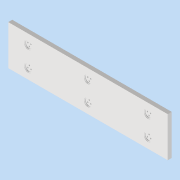
# Autodesk Inventor part: Platt oben
Saved by Autodesk Inventor 2021 (Build 250183000, 183)
## iProperties
Created: 2024-03-13
Part Number: Platt oben
Material: Generic
Document SubType Name: Modeling
Designer: Nokia
Density: 1 g/cm^3
Appearance: Smooth - Ash
Mass: 3100.69 g
Surface Area: 3710.93 cm^2
Volume: 3100.69 cm^3
Author: Nokia
Autodesk Inventor part; units mm, degrees
ref_plane "YZ Plane" through (0, 0, 0) normal (1, 0, 0) x (0, 1, 0)
ref_plane "XZ Plane" through (0, 0, 0) normal (0, 1, 0) x (-1, 0, 0)
ref_plane "XY Plane" through (0, 0, 0) normal (0, 0, 1) x (1, 0, 0)
sketch "Sketch1" plane through (0, 0, 0) normal (0, 0, 1) x (1, 0, 0)
  line L0 (-400, -100) -> (-400, 100)
  line L1 (-400, 100) -> (400, 100)
  line L2 (400, 100) -> (400, -100)
  line L3 (400, -100) -> (-400, -100)
  point P0 (0, 0)
  dimension "d2" = 800
  dimension "d3" = 200
  constraints: 8 end point, 3 perpendicular
  measures "d2" distance of L0.end L1.end
  measures "d3" distance of L1.end L2.end
extrude "Extrusion1" add sketch "Sketch1" along normal blind 20
sketch "Sketch5" plane through (0, 0, 20) normal (0, 0, 1) x (1, 0, 0)
  line L0 (0, 0) -> (0, 50)
  circle A0 centre (0, 50) radius 17
  line L1 (0, 0) -> (-150, 0)
  line L2 (-150, 0) -> (-150, 100)
  line L3 (-400, 100) -> (400, 100)
  circle A1 centre (0, -50) radius 17
  circle A2 centre (-300, 50) radius 17
  circle A3 centre (-300, -50) radius 17
  circle A4 centre (300, 50) radius 17
  circle A5 centre (300, -50) radius 17
  circle A6 centre (0, 50) radius 20
  circle A7 centre (0, -50) radius 20
  circle A8 centre (-300, 50) radius 20
  circle A9 centre (-300, -50) radius 20
  circle A10 centre (300, -50) radius 20
  circle A11 centre (300, 50) radius 20
  dimension "d18" = 50
  dimension "d19" = 34
  dimension "d20" = 150
  dimension "d43" = 40
  constraints: 12 centre point, 10 symmetric about line, 8 end point, 2 coincident, 1 horizontal, 1 perpendicular, 1 point on line, 1 vertical, 10 other
  measures "d18" distance of L0.start L0.end
  measures "d19" diameter of A0
  measures "d20" distance of L0.start L1.end
  measures "d43" diameter of A6
extrude "Extrusion4" cut sketch "Sketch5" against normal blind 6 contours A0 | A1 | A2 | A3 | A4 | A5
sketch "Sketch6" plane through (0, 0, 0) normal (0, 0, -1) x (-1, 0, 0)
  line L0 (0, 0) -> (0, 50)
  circle A0 centre (0, 50) radius 20
  line L1 (0, 0) -> (-150, 0)
  line L2 (-150, 0) -> (-150, 100)
  line L3 (-400, 100) -> (400, 100)
  circle A1 centre (0, -50) radius 20
  circle A2 centre (-300, 50) radius 20
  circle A3 centre (-300, -50) radius 20
  circle A4 centre (300, 50) radius 20
  circle A5 centre (300, -50) radius 20
  circle A6 centre (0, 50) radius 15
  circle A7 centre (0, 41) radius 3.5
  circle A8 centre (7.7942, 54.5) radius 3.5
  circle A9 centre (-7.7942, 54.5) radius 3.5
  circle A10 centre (0, -50) radius 15
  circle A11 centre (0, -41) radius 3.5
  circle A12 centre (7.7942, -54.5) radius 3.5
  circle A13 centre (-7.7942, -54.5) radius 3.5
  circle A14 centre (-300, 50) radius 15
  circle A15 centre (-300, 41) radius 3.5
  circle A16 centre (-307.7942, 54.5) radius 3.5
  circle A17 centre (-292.2058, 54.5) radius 3.5
  circle A18 centre (-307.7942, -54.5) radius 3.5
  circle A19 centre (-300, -41) radius 3.5
  circle A20 centre (-292.2058, -54.5) radius 3.5
  circle A21 centre (-300, -50) radius 15
  circle A22 centre (300, -50) radius 15
  circle A23 centre (292.2058, -54.5) radius 3.5
  circle A24 centre (300, -41) radius 3.5
  circle A25 centre (307.7942, -54.5) radius 3.5
  circle A26 centre (300, 41) radius 3.5
  circle A27 centre (292.2058, 54.5) radius 3.5
  circle A28 centre (307.7942, 54.5) radius 3.5
  circle A29 centre (300, 50) radius 15
  dimension "d23" = 50
  dimension "d24" = 40
  dimension "d25" = 150
  dimension "d28" = 30
  dimension "d30" = 7
  dimension "d33" = 360
  dimension "d42" = 9
  constraints: 30 centre point, 25 symmetric about line, 8 end point, 2 coincident, 1 horizontal, 1 perpendicular, 1 point on line, 1 vertical, 32 other
  measures "d23" distance of L0.start L0.end
  measures "d24" diameter of A0
  measures "d25" distance of L0.start L1.end
  measures "d28" diameter of A6
  measures "d30" diameter of A7
  measures "d42" distance of A7.centre L0.end
extrude "Extrusion5" cut sketch "Sketch6" against normal blind 8 contours A7 L0 | L0 A7 | A0 | A1 | A2 | A3 | A4 | A5 | A6 | A8 | A9 | A10 | A11 | A12 | A13 | A14 | A15 | A16 | A17 | A18 | A19 | A20 | A21 | A22 | A23 | A24 | A25 | A26 | A27 | A28 | A29
hole "Hole1" at (-307.7942, -54.5, 0) at (-292.2058, -54.5, 0) at (-300, -41, 0) at (-300, 41, 0) at (-307.7942, 54.5, 0) at (-292.2058, 54.5, 0) at (-7.7942, -54.5, 0) at (7.7942, -54.5, 0) at (0, -41, 0) at (-7.7942, 54.5, 0) at (0, 41, 0) at (7.7942, 54.5, 0) at (292.2058, -54.5, 0) at (300, -41, 0) at (307.7942, -54.5, 0) at (292.2058, 54.5, 0) at (300, 41, 0) at (307.7942, 54.5, 0) direction (0, 0, 1) diameter 7 depth 55
extrude "Extrusion6" cut sketch "Sketch5" against normal blind 2
body "Solid1"
